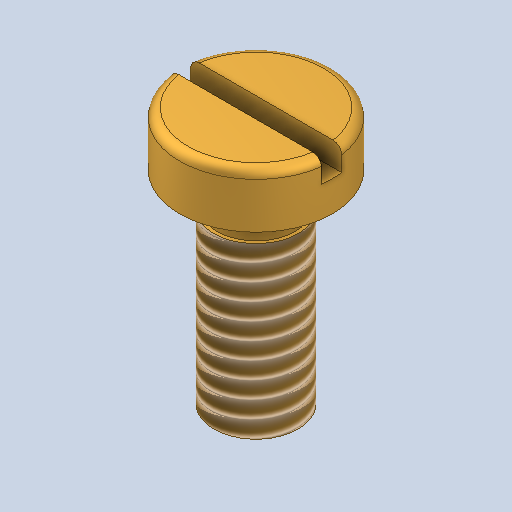
# Autodesk Inventor part: Screw-CheeseHead-Brass-M2.5x08
Saved by Autodesk Inventor 2026 (Build 300175050, 175E)
## iProperties
Created: 2023-08-07
Part Number: Screw-CheeseHead-Brass-M2.5x08
Material: Brass, Soft Yellow
Document SubType Name: Modeling
Designer: schanen
Density: 8.47 g/cm^3
Appearance: Brass - Satin
Author: schanen
Autodesk Inventor part; units mm, degrees
ref_plane "YZ Plane" through (0, 0, 0) normal (1, 0, 0) x (0, 1, 0)
ref_plane "XZ Plane" through (0, 0, 0) normal (0, 1, 0) x (-1, 0, 0)
ref_plane "XY Plane" through (0, 0, 0) normal (0, 0, 1) x (1, 0, 0)
sketch "Sketch1" plane through (0, 0, 0) normal (0, 0, 1) x (1, 0, 0)
  line L0 (0, 0) -> (-1.25, 0)
  line L1 (-1.25, 0) -> (-1.25, 5)
  line L2 (-1.25, 5) -> (-1.15, 5)
  line L3 (-1.15, 5) -> (-1.15, 6)
  line L4 (-1.15, 6) -> (-2.25, 6)
  line L5 (-2.25, 6) -> (-2.25, 7.6)
  line L6 (-2.25, 7.6) -> (0, 7.6)
  line L7 (0, 7.6) -> (0, 0)
  dimension "d0" = 1.6
  dimension "d1" = 2.25
  dimension "d2" = 1.25
  dimension "d3" = 0.1
  dimension "d4" = 1
  dimension "d5" = 7.6
  dimension "d6" = 90
  constraints: 16 end point, 6 perpendicular, 1 vertical
  measures "d0" distance between parallel lines of L4 L6
  measures "d1" distance of L5.end L6.end
  measures "d2" distance between parallel lines of L7 L1
  measures "d3" distance between parallel lines of L3 L1
  measures "d4" distance between parallel lines of L2 L4
  measures "d5" distance of L6.end L0.start
  measures "d6" angle of L7 L0
revolve "Revolution1" add sketch "Sketch1" angle 360 about axis through (0, 7.6, 0) along (0, -1, 0)
thread "Thread1" size "M3x0.5" class "6g" standard "ANSI Metric M Profile" length 27
sketch "Sketch2" plane through (0, 7.6, 0) normal (0, 1, 0) x (1, 0, 0)
  line L0 (5, 0.3) -> (-5, 0.3)
  line L1 (-5, 0.3) -> (-5, -0.3)
  line L2 (-5, -0.3) -> (5, -0.3)
  line L3 (5, -0.3) -> (5, 0.3)
  line L4 (5, 0.3) -> (-5, -0.3) construction
  line L5 (-5, 0.3) -> (5, -0.3) construction
  point P0 (0, 0)
  dimension "d10" = 10
  dimension "d11" = 0.6
  constraints: 12 end point, 2 midpoint, 2 parallel, 1 horizontal, 1 perpendicular
  measures "d10" distance of L2.end L1.end
  measures "d11" distance of L1.end L0.end
fillet "Fillet1" radius 0.25 1 edges at (2.25, 7.6, 0)
extrude "Extrusion2" cut sketch "Sketch2" against normal blind 0.7
fillet "Fillet2" radius 0.3 1 edges at (1.15, 6, 0)
body "Solid1"
